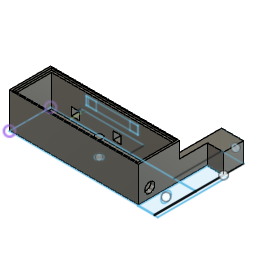
GaszählerSensor_v1 (Autodesk Fusion 360 design; units mm, degrees)
Autodesk Fusion 360 part; units mm, degrees
sketch "Skizze1" plane through (0, 0, 0) normal (0, 1, 0) x (1, 0, 0)
  line L0 (63.1665, -18) -> (63.1665, -42)
  line L1 (0.1665, -42) -> (0.1665, -35)
  line L2 (30.1665, -42) -> (52.1665, -42)
  line L3 (63.1665, -28) -> (63.1665, -62.6883)
  line L4 (0.1665, -42) -> (30.1665, -42)
  line L5 (52.1665, -18) -> (63.1665, -18)
  line L6 (52.1665, -42) -> (63.1665, -42)
  line L7 (0.1665, -35) -> (30.1665, -35)
  line L8 (0.1665, -35) -> (0.1665, -36.5)
  line L9 (63.1665, -42) -> (63.1665, -62.6883)
  line L10 (30.1665, -35) -> (30.1665, -42)
  line L11 (-1.8335, -36.5) -> (-1.8335, -35)
  line L12 (0.1665, -36.5) -> (-1.8335, -36.5)
  line L13 (52.1665, -42) -> (52.1665, -18)
  line L14 (-1.8335, -35) -> (0.1665, -35)
  line L15 (63.1665, -62.6883) -> (-10, -62.6883)
  line L16 (-10, -62.6883) -> (-10, -42)
  line L17 (-10, -42) -> (63.1665, -42)
  line L18 (63.1665, -42) -> (63.1665, -62.6883)
  dimension "d1" = 30
  dimension "d3" = 24
  dimension "d4" = 7
  dimension "d5" = 2
  dimension "d6" = 1.5
  dimension "d8" = 11
  dimension "d34" = 52
  constraint vertical L1
  constraint perpendicular L1 L7
  constraint perpendicular L7 L10
  constraint perpendicular L2 L10
  constraint perpendicular L2 L13
  constraint perpendicular L5 L13
  constraint perpendicular L0 L2
  constraint perpendicular L2 L9
  constraint horizontal L14
  constraint vertical L8
  constraint horizontal L12
  constraint vertical L11
  constraint coincident L8.end L1
  constraint perpendicular L4 L10
  constraint perpendicular L0 L6
  constraint vertical L3
  constraint horizontal L15
  constraint vertical L16
  constraint horizontal L17
  constraint vertical L18
  constraint coincident L1.start L17
  constraint coincident L4.start L1
  measures "d1" distance of L1.end L7.end
  measures "d3" distance of L5.start L2.end
  measures "d4" distance of L1.start L1.end
  measures "d5" distance of L1.end L11.end
  measures "d6" distance of L11.start L11.end
  measures "d8" distance of L5.start L0.start
  measures "d34" distance of L1 L13
extrude "Extrusion1" add sketch "Skizze1" along normal blind 10 contours L1 L4 L7 L8 L10 L17 | L1 L8 L11 L12 L14 makes body 1
extrude "Extrusion2" add sketch "Skizze1" along normal blind 10 separate body contours L0 L3 L5 L6 L13 L17 makes body 2
extrude "Extrusion22" add sketch "Skizze1" along normal blind 18 contours L2 L3 L4 L6 L9 L15 L16 L17 L18 bodies 1 2
extrude "Extrusion3" add sketch "Skizze1" along normal blind 10 contours L2 L3 L4 L6 L9 L15 L16 L17 L18 bodies 1
chamfer "Fase1" distance 2 angle 45 3 edges at (14.1665, 10, 35) (14.1665, 0, 35) (30.1665, 5, 35) on bodies 1
sketch "Skizze3" plane through (0, 0, 35) normal (0, 0, -1) x (-1, 0, 0)
  line L0 (-28.1665, 2) -> (1.8335, 2)
  line L1 (1.8335, 2) -> (1.8335, 8)
  line L2 (1.8335, 8) -> (-28.1665, 8)
  line L3 (-28.1665, 8) -> (-28.1665, 2)
  line L4 (-27, 7) -> (-1, 7)
  line L5 (-1, 7) -> (-1, 3)
  line L6 (-1, 3) -> (-27, 3)
  line L7 (-27, 3) -> (-27, 7)
  line L8 (-27, 7) -> (-23, 7)
  line L9 (-23, 7) -> (-23, 3)
  line L10 (-23, 3) -> (-27, 3)
  line L11 (-27, 3) -> (-27, 7)
  line L12 (-6, 7) -> (-1, 7)
  line L13 (-1, 7) -> (-1, 3)
  line L14 (-1, 3) -> (-6, 3)
  line L15 (-6, 3) -> (-6, 7)
  line L16 (-2, 7) -> (-2, 3)
  constraint horizontal L4
  constraint vertical L5
  constraint horizontal L6
  constraint vertical L7
  constraint horizontal L8
  constraint vertical L9
  constraint horizontal L10
  constraint vertical L11
  constraint coincident L6 L9.end
  constraint horizontal L12
  constraint vertical L13
  constraint horizontal L14
  constraint vertical L15
  constraint coincident L6 L5.end
  constraint coincident L4 L12.start
  constraint coincident L12 L16.start
  constraint coincident L14 L16.end
extrude "Extrusion4" cut sketch "Skizze3" against normal blind 3 contours L4 L6 L9 L15 bodies 1
extrude "Extrusion9" cut sketch "Skizze3" against normal blind 9 contours L4 L6 L7 L8 L9 L10 L11 | L4 L6 L12 L14 L15 L16 bodies 1
sketch "Skizze4" plane through (0, 0, 18) normal (0, 0, -1) x (-1, 0, 0)
  line L0 (-63.1665, 0) -> (-52.1665, 0)
  line L1 (-52.1665, 0) -> (-52.1665, 10)
  line L2 (-52.1665, 10) -> (-63.1665, 10)
  line L3 (-63.1665, 10) -> (-63.1665, 0)
  circle A0 centre (-59.1665, 5) radius 1.5
  dimension "d23" = 3
  dimension "d77" = 7
  measures "d23" diameter of A0
  measures "d77" distance of L1 A0.centre
extrude "Extrusion6" cut sketch "Skizze4" against normal blind 7 contours A0 bodies 1
sketch "Skizze5" plane through (63.1665, 0, 0) normal (1, 0, 0) x (0, 0, -1)
  circle A0 centre (-57, 5) radius 2.5
  dimension "d42" = 5
  measures "d42" diameter of A0
extrude "Extrusion7" cut sketch "Skizze5" against normal blind 17 bodies 1
sketch "Skizze15" plane through (0, 0, 0) normal (0, 1, 0) x (1, 0, 0)
  line L0 (65, -63) -> (55, -63)
  line L1 (55, -63) -> (55, -28)
  line L2 (55, -28) -> (65, -28)
  line L3 (65, -28) -> (65, -63)
  line L4 (-10, -42) -> (-10, -62.6883) construction
  constraint horizontal L0
  constraint vertical L1
  constraint horizontal L2
  constraint vertical L3
extrude "Extrusion23" cut sketch "Skizze15" along normal blind 20 bodies 1
sketch "Skizze16" plane through (0, 0, 0) normal (0, 1, 0) x (1, 0, 0)
  line L0 (54, -62, 18) -> (-9, -62, 18)
  line L1 (-9, -62, 18) -> (-9, -42.5, 18)
  line L2 (-9, -42.5, 18) -> (54, -42.5, 18)
  line L3 (54, -42.5, 18) -> (54, -62, 18)
  line L4 (53, -61, 18) -> (-8, -61, 18)
  line L5 (-8, -61, 18) -> (-8, -43.5, 18)
  line L6 (-8, -43.5, 18) -> (53, -43.5, 18)
  line L7 (53, -43.5, 18) -> (53, -61, 18)
  line L8 (-9, -67) -> (-9, -40)
  dimension "d98" = 63
  dimension "d99" = 19.5
  dimension "d100" = 17.5
  dimension "d101" = 61
extrude "Extrusion25" cut sketch "Skizze16" against normal blind 17 contours L4 L5 L6 L7 in plane through (0, 18, 0) normal (0, 1, 0) bodies 1
extrude "Extrusion26" cut sketch "Skizze16" against normal blind 1 contours L0 L1 L2 L3 in plane through (0, 18, 0) normal (0, 1, 0) bodies 1
fillet "Abrundung2" radius 1 1 edges at (52.1665, 5, 42) on bodies 1
chamfer "Fase11" distance 0.3 angle 45 3 edges at (52.1665, 0, 29.5) (51.8736, 0, 41.7071) (40.6665, 0, 42) on bodies 1
ref_plane "Arbeitsebene5" through (26.5832, 1, 52.3441) normal (0, 1, 0) x (1, 0, 0)
sketch "Skizze18" plane through (26.5832, 1, 52.3441) normal (0, 1, 0) x (1, 0, 0)
  circle A0 centre (-1.6, -0.2) radius 1.75
  dimension "d126" = 3.5
  measures "d126" diameter of A0
extrude "Extrusion33" add sketch "Skizze18" along normal blind 9 bodies 1
chamfer "Fase15" distance 1 angle 45 1 edges at (23.3517, 1, 51.9113) on bodies 1
chamfer "Fase16" distance 0.3 angle 45 4 edges at (-10, 0, 52.3441) (22.5, 0, 62.6883) (-4.9168, 0, 42) (55, 0, 45.3441) on bodies 1
named bodies: "Gehäuse"
